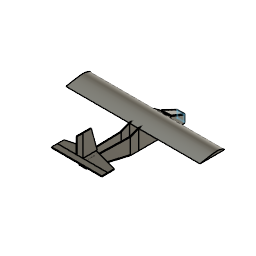
Apex 0 (Autodesk Fusion 360 archive; units mm, degrees)
design "Body"
part number: 2026-03-20-19-53-51-322
Autodesk Fusion 360 part; units mm, degrees
sketch "Body_top_1" plane through (0, 0, 0) normal (0, 0, 1) x (1, 0, 0)
  line L0 (0, 0) -> (25, 0)
  line L1 (0, 0) -> (-25, 0)
  line L2 (0, -90) -> (30, -90)
  line L3 (0, -90) -> (-30, -90)
  line L4 (25, 0) -> (30, -90)
  line L5 (-25, 0) -> (-30, -90)
  constraint coincident L0.start L1.start
  constraint horizontal L0
  constraint parallel L0 L1
extrude "Extrude1" add sketch "Body_top_1" along normal blind 5 contours L0 L1 L2 L3 L4 L5 picked at (-18.333333, -60) makes body 1
sketch "Body_side_1" plane through (0, 0, 0) normal (1, 0, 0) x (0, 1, 0)
  line L0 (0, 70) -> (-90, 70)
  line L1 (0, 70) -> (0, 110)
  line L2 (-90, 70) -> (-90, 150)
  line L3 (0, 110) -> (-90, 150)
  constraint horizontal L0
  constraint perpendicular L0 L1
  constraint perpendicular L0 L2
extrude "Extrude2" add sketch "Body_side_1" along normal blind 5 separate body contours L0 L1 L2 L3 picked at (-60, 110) makes body 2
move_body "Align1" bodies 2 to x (0.99846035, -0.05547002, 0) y (0.05547002, 0.99846035, 0) z (0, 0, 1) at (-24.919234, 1.453793, -65)
move_face "MoveFace1" by (0, -5, 0) 1 faces at (-24.919234, -58.638728, 71.666667) on bodies 2
move_body "Move1" bodies 2 to x (1, 0, 0) y (0, 1, 0) z (0, 0, 1) at (0, -1, 0)
copy_body "CopyPasteBodies1" bodies 2 makes body 3
move_body "Move2" bodies 3 to x (1, 0, 0) y (0, 1, 0) z (0, 0, 1) at (0, 0, 0)
move_body "Move3" bodies 2 to x (1, 0, 0) y (0, 1, 0) z (0, 0, 1) at (45, 0, 0)
move_body "Align2" bodies 2 to x (0.99384615, 0.11076923, 0) y (-0.11076923, 0.99384615, 0) z (0, 0, 1) at (0.075864, -2.504332, 0)
sketch "Body_top_2" plane through (0, 0, 0) normal (0, 0, 1) x (1, 0, 0)
  line L0 (-27.217662, -143.923697) -> (32.782338, -143.923697)
  line L1 (-27.217662, -143.923697) -> (-27.217662, -183.923697)
  line L2 (32.782338, -143.923697) -> (32.782338, -183.923697)
  line L3 (-27.217662, -183.923697) -> (32.782338, -183.923697)
  constraint horizontal L0
  constraint perpendicular L0 L1
  constraint perpendicular L0 L2
extrude "Extrude3" add sketch "Body_top_2" along normal blind 5 separate body contours L0 L1 L2 L3 picked at (-7.217662, -157.25703) makes body 4
move_body "Align3" bodies 4 to x (1, 0, 0) y (0, 1, 0) z (0, 0, 1) at (0, 53.923697, 0)
move_body "Align4" bodies 4 to x (1, 0, 0) y (0, 1, 0) z (0, 0, 1) at (-2.782338, 0, 0)
sketch "Body_side_2" plane through (0, 0, 0) normal (1, 0, 0) x (0, 1, 0)
  line L0 (0, -175) -> (0, -95)
  line L1 (0, -175) -> (-40, -175)
  line L2 (-40, -175) -> (-40, -65)
  line L3 (0, -95) -> (-40, -65)
  constraint vertical L0
  constraint perpendicular L0 L1
  constraint perpendicular L1 L2
extrude "Extrude4" add sketch "Body_side_2" along normal blind 5 separate body contours L0 L1 L2 L3 picked at (-26.666667, -111.666667) makes body 5
move_body "Align5" bodies 5 to x (1, 0, 0) y (0, 1, 0) z (0, 0, 1) at (-30, 0, 180)
move_body "Move4" bodies 5 to x (1, 0, 0) y (0, 1, 0) z (0, 0, 1) at (0, -90, 0)
copy_body "CopyPasteBodies2" bodies 5 makes body 6
move_body "Move5" bodies 6 to x (1, 0, 0) y (0, 1, 0) z (0, 0, 1) at (60, 0, 0)
move_body "Move6" bodies 6 to x (1, 0, 0) y (0, 1, 0) z (0, 0, 1) at (-5, 0, 0)
sketch "Body_top_3" plane through (0, 0, 0) normal (0, 0, 1) x (1, 0, 0)
  line L0 (-26.642094, -181.47513) -> (33.357906, -181.47513)
  line L1 (-26.642094, -181.47513) -> (-26.642094, -331.47513)
  line L2 (33.357906, -181.47513) -> (33.357906, -331.47513)
  line L3 (-26.642094, -331.47513) -> (33.357906, -331.47513)
  constraint horizontal L0
  constraint perpendicular L0 L1
  constraint perpendicular L0 L2
  constraint perpendicular L1 L3
extrude "Extrude5" add sketch "Body_top_3" along normal blind 5 separate body contours L0 L1 L2 L3 picked at (-6.642094, -231.47513) makes body 7
move_body "Align6" bodies 7 to x (1, 0, 0) y (0, 1, 0) z (0, 0, 1) at (-3.357906, 51.47513, 0)
sketch "Body_side_3" plane through (0, 0, 0) normal (1, 0, 0) x (0, 1, 0)
  line L0 (0, -200) -> (-150, -200)
  line L1 (0, -200) -> (0, -90)
  line L2 (-150, -200) -> (-150, -90)
  line L3 (0, -90) -> (-150, -90)
  constraint horizontal L0
  constraint perpendicular L0 L1
  constraint perpendicular L0 L2
extrude "Extrude6" add sketch "Body_side_3" along normal blind 5 separate body contours L0 L1 L2 L3 picked at (-50, -163.333333) makes body 8
move_body "Align7" bodies 8 to x (1, 0, 0) y (0, 1, 0) z (0, 0, 1) at (-30, 0, 205)
move_body "Move7" bodies 8 to x (1, 0, 0) y (0, 1, 0) z (0, 0, 1) at (0, -130, 0)
copy_body "CopyPasteBodies3" bodies 8 makes body 9
move_body "Move8" bodies 9 to x (1, 0, 0) y (0, 1, 0) z (0, 0, 1) at (55, 0, 0)
sketch "Body_top_4" plane through (0, 0, 0) normal (0, 0, 1) x (1, 0, 0)
  line L0 (-61.088052, -351.843683) -> (-1.088052, -351.843683)
  line L1 (-61.088052, -351.843683) -> (-61.088052, -401.843683)
  line L2 (-1.088052, -351.843683) -> (-1.088052, -401.843683)
  line L3 (-61.088052, -401.843683) -> (-1.088052, -401.843683)
  constraint horizontal L0
  constraint perpendicular L0 L1
  constraint perpendicular L0 L2
extrude "Extrude7" add sketch "Body_top_4" along normal blind 5 separate body contours L0 L1 L2 L3 picked at (-41.088052, -385.177016) makes body 10
move_body "Align8" bodies 10 to x (1, 0, 0) y (0, 1, 0) z (0, 0, 1) at (0, 71.843683, 0)
move_body "Align9" bodies 10 to x (1, 0, 0) y (0, 1, 0) z (0, 0, 1) at (31.088052, 0, 0)
sketch "Body_side_4" plane through (0, 0, 0) normal (1, 0, 0) x (0, 1, 0)
  line L0 (0, -214.93215) -> (-50, -214.93215)
  line L1 (0, -214.93215) -> (0, -104.93215)
  line L2 (-50, -214.93215) -> (-50, -124.93215)
  line L3 (0, -104.93215) -> (-50, -124.93215)
  constraint horizontal L0
  constraint perpendicular L0 L1
  constraint perpendicular L0 L2
extrude "Extrude8" add sketch "Body_side_4" along normal blind 5 separate body contours L0 L1 L2 L3 picked at (-16.666667, -148.265484) makes body 11
move_body "Align10" bodies 11 to x (1, 0, 0) y (0, 1, 0) z (0, 0, 1) at (-30, 0, 219.93215)
move_body "Move9" bodies 11 to x (1, 0, 0) y (0, 1, 0) z (0, 0, 1) at (0, -280, 0)
copy_body "CopyPasteBodies4" bodies 11 makes body 12
move_body "Move10" bodies 12 to x (1, 0, 0) y (0, 1, 0) z (0, 0, 1) at (55, 0, 0)
sketch "Body_top_5" plane through (0, 0, 0) normal (0, 0, 1) x (1, 0, 0)
  line L0 (-20.138143, -488.014323) -> (39.861857, -488.014323)
  line L1 (9.861857, -748.014323) -> (32.361857, -748.014323)
  line L2 (9.861857, -748.014323) -> (-12.638143, -748.014323)
  line L3 (39.861857, -488.014323) -> (32.361857, -748.014323)
  line L4 (-20.138143, -488.014323) -> (-12.638143, -748.014323)
  constraint horizontal L0
extrude "Extrude9" add sketch "Body_top_5" along normal blind 5 separate body contours L0 L1 L2 L3 L4 picked at (9.861857, -574.680989) makes body 13
move_body "Align11" bodies 13 to x (1, 0, 0) y (0, 1, 0) z (0, 0, 1) at (0, 158.014323, 0)
move_body "Align12" bodies 13 to x (1, 0, 0) y (0, 1, 0) z (0, 0, 1) at (-9.861857, 0, 0)
move_body "Move11" bodies 13 to x (1, 0, 0) y (0, 0.9781476, -0.20791169) z (0, 0.20791169, 0.9781476) at (0, -8.25085, -68.501596)
sketch "Body_side_5" plane through (0, 0, 0) normal (1, 0, 0) x (0, 1, 0)
  line L0 (-584.335649, 59.097627) -> (-330.000005, 5)
  line L1 (-330.000005, 5) -> (-330.000005, 95.000001)
  line L2 (-330.000005, 95.000001) -> (-584.297672, 95.000001)
  line L3 (-584.297672, 95.000001) -> (-584.335649, 59.097627)
  constraint perpendicular L1 L2
extrude "Extrude10" add sketch "Body_side_5" along normal blind 5 separate body contours L0 L1 L2 L3 picked at (-414.778553, 53.032543) makes body 14
move_body "Move12" bodies 14 to x (1, 0, 0) y (0, 1, 0) z (0, 0, 1) at (-30, 0, 0)
move_body "Align13" bodies 14 to x (0.99958421, 0.02820365, -0.00599692) y (-0.02820282, 0.9996022, 0.00022343) z (0.00600083, -0.0000542, 0.99998199) at (-9.350966, 0.767962, -0.117321)
move_body "Align14" bodies 13 to x (1, 0, 0) y (0, 1, 0) z (0, 0, 1) at (-0.001559, 0.052851, -0.011234)
copy_body "CopyPasteBodies5" bodies 14 makes body 15
move_body "Move13" bodies 15 to x (1, 0, 0) y (0, 1, 0) z (0, 0, 1) at (40, 0, 0)
move_body "Move14" bodies 15 to x (1, 0, 0) y (0, 1, 0) z (0, 0, 1) at (0, 0, 60)
move_body "Align15" bodies 15 to x (0.99833718, -0.05638467, 0.01198493) y (0.05638467, 0.99840906, 0.00033816) z (-0.01198493, 0.00033816, 0.99992812) at (34.039921, -12.104741, -57.427048)
move_body "Align16" bodies 15 to x (1, 0, 0) y (0, 1, 0) z (0, 0, 1) at (0.361632, 12.26262, -2.6065)
move_body "Align17" bodies 14 to x (1, 0, 0) y (0, 1, 0) z (0, 0, 1) at (0.001559, -0.052851, 0.011234)
move_body "Align18" bodies 13 to x (1, 0, 0) y (0, 1, 0) z (0, 0, 1) at (0.001559, -0.052851, 0.011234)
move_body "Align19" bodies 10 to x (1, 0, 0) y (0, 0, 1) z (0, -1, 0) at (0, -325, 310)
move_body "Align20" bodies 15 to x (1, 0, 0) y (0, 1, 0) z (0, 0, 1) at (0.001559, -0.052851, 0.011234)
move_body "Align21" bodies 10 to x (1, 0, 0) y (0, 1, 0) z (0, 0, 1) at (0, 45, 25)
move_body "Align22" bodies 10 to x (1, 0, 0) y (0, 1, 0) z (0, 0, 1) at (0, -45, -50)
move_body "Move15" bodies 10 to x (1, 0, 0) y (0, 0, 1) z (0, -1, 0) at (0, -375, 285)
move_body "Align23" bodies 10 to x (1, 0, 0) y (0, 1, 0) z (0, 0, 1) at (0, 50, 45)
sketch "Elevator" plane through (0, 0, 0) normal (0, 0, 1) x (1, 0, 0)
  line L0 (-126.599306, -1017.483313) -> (173.400694, -1017.483313)
  line L1 (-126.599306, -1017.483313) -> (-126.599306, -982.483313)
  line L2 (173.400694, -1017.483313) -> (173.400694, -982.483313)
  line L3 (-126.599306, -982.483313) -> (173.400694, -982.483313)
  line L4 (-125, -950) -> (175, -950)
  line L5 (175, -950) -> (175, -910)
  line L6 (-125, -950) -> (-125, -910)
  line L7 (-125, -910) -> (25, -870)
  line L8 (175, -910) -> (25, -870)
  constraint horizontal L0
  constraint perpendicular L0 L1
  constraint perpendicular L0 L2
  constraint perpendicular L2 L3
  constraint horizontal L4
  constraint perpendicular L4 L5
  constraint perpendicular L4 L6
extrude "Extrude11" add sketch "Elevator" along normal blind 5 separate body contours L0 L1 L2 L3 | L4 L5 L6 L7 L8 picked at (-26.599306, -994.149979) picked at (25, -923.333333) makes body 16 at (25, -923.333333, 0) makes body 17 at (-26.599306, -994.149979, 0)
move_body "Move16" bodies 16 to x (1, 0, 0) y (0, 1, 0) z (0, 0, 1) at (-25, 370, 0)
move_body "Align25" bodies 16 to x (1, 0, 0) y (0, 1, 0) z (0, 0, 1) at (0, -5.357935, 54.166302)
move_body "Move17" bodies 16 to x (1, 0, 0) y (0, 1, 0) z (0, 0, 1) at (0, 0, 40)
move_body "Move18" bodies 16 to x (1, 0, 0) y (0, 1, 0) z (0, 0, 1) at (0, 0, 1)
move_body "Align26" bodies 17 to x (1, 0, 0) y (0, 1, 0) z (0, 0, 1) at (0, 397.125378, 95.166302)
move_body "Align27" bodies 17 to x (1, 0, 0) y (0, 1, 0) z (0, 0, 1) at (-23.400694, 0, 0)
sketch "Rudder" plane through (0, 0, 0) normal (1, 0, 0) x (0, 1, 0)
  line L0 (0, -481.912283) -> (-85, -481.912283)
  line L1 (-85, -481.912283) -> (-85, -351.912283)
  line L2 (-85, -351.912283) -> (-35, -351.912283)
  line L3 (-35, -351.912283) -> (0, -481.912283)
  line L4 (-160.825661, -446.912283) -> (-160.825661, -351.912283)
  line L5 (-125.825661, -481.912283) -> (-125.825661, -351.912283)
  line L6 (-160.825661, -351.912283) -> (-125.825661, -351.912283)
  line L7 (-125.825661, -481.912283) -> (-160.825661, -446.912283)
  line L8 (-125.825661, -481.912283) -> (-76.328187, -481.912283) construction
  constraint horizontal L0
  constraint perpendicular L0 L1
  constraint perpendicular L1 L2
  constraint perpendicular L5 L6
  constraint horizontal L8
extrude "Extrude12" add sketch "Rudder" along normal blind 5 separate body contours L0 L1 L2 L3 | L4 L5 L6 L7 picked at (-40, -438.578949) picked at (-137.492328, -426.912283) makes body 18 at (0, -40, -438.578949) makes body 19 at (0, -137.492328, -426.912283)
move_body "Align28" bodies 19 to x (1, 0, 0) y (0, 1, 0) z (0, 0, 1) at (0, 40.825661, 0)
move_body "Move19" bodies 18 19 to x (1, 0, 0) y (0, 1, 0) z (0, 0, 1) at (-2.5, 0, 590)
move_body "Move20" bodies 19 18 to x (1, 0, 0) y (0, 1, 0) z (0, 0, 1) at (0, 0, 80)
move_body "Align29" bodies 18 to x (1, 0, 0) y (0, 1, 0) z (0, 0, 1) at (0, 0, -87.921416)
move_body "Align30" bodies 19 to x (1, 0, 0) y (0, 1, 0) z (0, 0, 1) at (0, -500.357935, -87.921416)
move_body "Move21" bodies 18 to x (1, 0, 0) y (0, 1, 0) z (0, 0, 1) at (0, -500, 0)
combine "Combine1" operation add target body 3 tool bodies 2 makes body 20 at (23.310991, -59.736622, 43.520799)
combine "Combine2" operation add target body 1 tool bodies 3 20
combine "Combine3" operation add target body 5 tool bodies 4 6
combine "Combine4" operation add target body 8 tool bodies 7 9
combine "Combine5" operation add target body 11 tool bodies 10 12
combine "Combine6" operation add target body 15 tool bodies 14 13
sketch "Sketch14" plane through (0, 0, 0) normal (1, 0, 0) x (0, 1, 0)
  line L0 (75.000001, -200.000003) -> (-70, -200.000003)
  spline S0 degree 5 poles (75.000001, -200.000003) (75.279178, -199.515697) (75.721339, -198.576902) (76.035905, -197.258199) (75.757574, -195.678868) (74.285311, -193.988377) (71.834885, -192.527139) (68.643766, -191.211222) (64.967502, -189.961604) (61.022722, -188.731986) (56.92536, -187.538324) (52.71994, -186.435656) (48.405752, -185.496332) (43.96272, -184.788919) (39.379986, -184.354289) (34.674753, -184.190557) (29.877299, -184.268681) (25.021748, -184.542754) (20.13458, -184.962216) (15.22423, -185.483037) (10.269736, -186.079626) (5.228274, -186.741204) (0.042903, -187.46796) (-5.349754, -188.267303) (-11.012095, -189.150238) (-16.997378, -190.127454) (-23.343573, -191.206273) (-30.076793, -192.391601) (-37.21327, -193.686293) (-44.761731, -195.091702) (-52.72546, -196.608121) (-59.428574, -197.909811) (-64.642036, -198.93566) (-68.20025, -199.641556) (-70, -200.000003) knots 0 0 0 0 0 0 0.03333333 0.06666667 0.1 0.13333333 0.16666667 0.2 0.23333333 0.26666667 0.3 0.33333333 0.36666667 0.4 0.43333333 0.46666667 0.5 0.53333333 0.56666667 0.6 0.63333333 0.66666667 0.7 0.73333333 0.76666667 0.8 0.83333333 0.86666667 0.9 0.93333333 0.96666667 1 1 1 1 1 1
  point P0 (20, -185.000003)
  point P1 (75, -195)
  point P2 (65.000001, -190.000003)
  point P3 (45.000001, -185.000003)
  point P4 (-10, -189)
  constraint horizontal L0
extrude "Extrude13" add sketch "Sketch14" along normal blind 800 separate body contours L0 S0 picked at (-0.986472, -196.226533) makes body 21
move_body "Align31" bodies 21 to x (1, 0, 0) y (0, 1, 0) z (0, 0, 1) at (-30, 0, 315.000003)
move_body "Move22" bodies 21 to x (1, 0, 0) y (0, 1, 0) z (0, 0, 1) at (-375, 0, 0)
move_body "Move23" bodies 21 to x (1, 0, 0) y (0, 1, 0) z (0, 0, 1) at (0, -210, 0)
sketch "Sketch15" plane through (0, 0, 0) normal (0, 1, 0) x (1, 0, 0)
  line L0 (19.974404, -42.785159) -> (-19.929131, -42.785159)
  line L1 (-19.929131, -42.785159) -> (-19.929131, -5)
  line L2 (-19.929131, -5) -> (20, -5)
  line L3 (20, -5) -> (19.974404, -42.785159)
  constraint horizontal L0
  constraint perpendicular L0 L1
  constraint perpendicular L1 L2
extrude "Extrude14" cut sketch "Sketch15" along normal blind 5 contours L0 L1 L2 L3 picked at (6.681758, -17.595053) bodies 1
extrude "Extrude15" cut sketch "Sketch15" against normal blind 5 contours L0 L1 L2 L3 picked at (6.681758, -17.595053) bodies 1
extrude "Extrude16" add sketch "Sketch15" against normal blind 5 contours L0 L1 L2 L3 picked at (6.681758, -17.595053) bodies 1
ref_plane "WorkPlane1" through (24.975092, -44.621041, 62.781199) normal (-0.02252851, 0.40551316, 0.91381155) x (0.05068914, -0.9124046, 0.40613847)
sketch "Sketch16" plane through (-0.872149, 15.698677, 35.376491) normal (-0.02252851, 0.40551316, 0.91381155) x (0.05068914, -0.9124046, 0.40613847)
  line L0 (18.206967, 24.951967) -> (116.519114, 24.951967)
  line L1 (116.519114, 24.951967) -> (114.000002, -35.000001)
  line L2 (114.000002, -35.000001) -> (15, -25)
  line L3 (15, -25) -> (18.206967, 24.951967)
  constraint horizontal L0
extrude "Extrude17" add sketch "Sketch16" along normal blind 5 draft -5 contours L0 L1 L2 L3 picked at (82.908694, 4.967978) bodies 1 8 11 15 21 5
